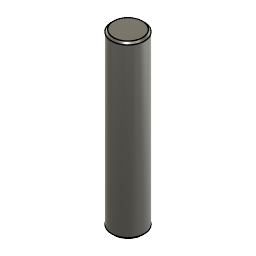
Parametric Pin (Autodesk Fusion 360 design; units mm, degrees)
part number: 5x26mm Pin
Autodesk Fusion 360 part; units mm, degrees
cylinder "CylinderPrimitive1" add diameter 5 height 26 placed x (1, 0, 0) y (0, 0, -1) z (0, 1, 0) at (0, 0, 0)
chamfer "Chamfer1" distance 0.3 angle 45 2 edges at (-2.3308, 26, 0.904) (-2.3308, 0, -0.904)
equation "Diameter = 5 mm"
equation "Length = 26 mm"
equation "d3 = Length"
equation "d4 = Diameter"
